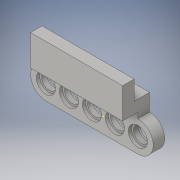
# Autodesk Inventor part: caster_pad
Saved by Autodesk Inventor 2016 (Build 200138000, 138)
## iProperties
Created: 2016-02-16
Part Number: caster_pad
Material: Generic
Document SubType Name: Modeling
Designer: jforce
Density: 1 g/cm^3
Appearance: Default
Author: jforce
## iProperties of the stored document caster_pad_3DPrint.ipt
Created: 2016-02-16
Part Number: caster_pad_3DPrint
Material: Generic
Document SubType Name: Modeling
Designer: jforce
Density: 1 g/cm^3
Appearance: Default
Author: jforce
Autodesk Inventor part; units mm, degrees
ref_plane "YZ Plane" through (0, 0, 0) normal (1, 0, 0) x (0, 1, 0)
ref_plane "XZ Plane" through (0, 0, 0) normal (0, 1, 0) x (-1, 0, 0)
ref_plane "XY Plane" through (0, 0, 0) normal (0, 0, 1) x (1, 0, 0)
sketch "Sketch1" plane through (0, 0, 0) normal (0, 0, 1) x (1, 0, 0)
  arc A0 (-15, 4) -> (-15, -4) centre (-15, 0) ccw
  line L0 (-5, -4) -> (-15, -4)
  line L1 (-3, 0) -> (-3, 5.2247) construction
  arc A1 (9, -4) -> (9, 4) centre (9, 0) ccw
  line L2 (-5, -4) -> (9, -4)
  line L3 (9, 8.4612) -> (-15, 8.4612)
  line L4 (-15, 8.4612) -> (-15, 4)
  line L5 (9, 4) -> (9, 8.4612)
  dimension "d11" = 4
  constraints: 12 end point, 4 point on circle, 3 symmetric about line, 2 centre point, 2 vertical, 1 other
  measures "d11" radius of A0
extrude "Extrusion1" add sketch "Sketch1" along normal blind 3
sketch "Sketch2" plane through (0, 0, 3) normal (0, 0, 1) x (1, 0, 0)
  arc A0 (-15, 4) -> (-15, -4) centre (-15, 0) ccw projected
  point P0 (0, 0)
hole "Hole1" at (-15, 0, 3) direction (0, 0, -1) diameter 4 depth 3 tip angle 118 counterbore diameter 5 counterbore depth 0.85
sketch "Sketch5" plane through (0, 0, 0) normal (0, 0, -1) x (-1, 0, 0)
  circle A0 centre (15, 0) radius 2 projected
  circle A1 centre (15, 0) radius 2.5
  point P0 (0, 0)
  constraints: 1 centre point, 1 coincident
extrude "Extrusion3" cut sketch "Sketch5" against normal blind 0.85
pattern_linear "Rectangular Pattern2" count 5 spacing 6 along (1, 0, 0) of "Extrusion3", "Hole1"
sketch "Sketch6" plane through (0, 0, 3) normal (0, 0, 1) x (1, 0, 0)
  point P0 (0, 0)
sketch "Sketch7" plane through (0, 0, 3) normal (0, 0, 1) x (1, 0, 0)
  line L0 (9, 4) -> (9, 8.4612) projected
  line L1 (-15, 8.4612) -> (9, 8.4612)
  line L2 (9, 8.4612) -> (9, 5.4612)
  line L3 (9, 5.4612) -> (-15, 5.4612)
  line L4 (-15, 5.4612) -> (-15, 8.4612)
  point P0 (0, 0)
  dimension "d24" = 3
  constraints: 8 end point, 2 parallel, 1 horizontal, 1 perpendicular, 1 point on line
  measures "d24" distance of L1.end L2.end
extrude "Extrusion4" add sketch "Sketch7" along normal blind 4
sketch "Sketch8" plane through (-15, 8.4612, 0) normal (0, 1, 0) x (1, 0, 0)
  line L0 (24, -3) -> (24, -7) projected
  line L1 (0, -7) -> (24, -7)
  line L2 (24, -7) -> (24, -4)
  line L3 (24, -4) -> (0, -4)
  line L4 (0, -4) -> (0, -7)
  point P0 (15, 0)
  dimension "d27" = 3
  constraints: 8 end point, 2 parallel, 1 horizontal, 1 perpendicular, 1 point on line
  measures "d27" distance of L2.end L1.end
extrude "Extrusion5" add sketch "Sketch8" along normal blind 5
body "Solid1"
